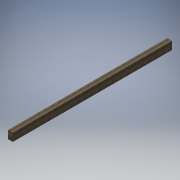
# Autodesk Inventor part: Bodenbalken
Saved by Autodesk Inventor 2017 (Build 210142000, 142)
## iProperties
Created: 2017-05-11
Part Number: Bodenbalken
Material: Generic
Document SubType Name: Modeling
Designer: Fake
Density: 1 g/cm^3
Appearance: Treibholz
Author: Fake
Autodesk Inventor part; units mm, degrees
ref_plane "YZ Plane" through (0, 0, 0) normal (1, 0, 0) x (0, 1, 0)
ref_plane "XZ Plane" through (0, 0, 0) normal (0, 1, 0) x (-1, 0, 0)
ref_plane "XY Plane" through (0, 0, 0) normal (0, 0, 1) x (1, 0, 0)
sketch "Skizze2" plane through (0, 0, 0) normal (0, 1, 0) x (-1, 0, 0)
  line L0 (30, 50) -> (-30, 50)
  line L1 (-30, 50) -> (-30, -50)
  line L2 (-30, -50) -> (30, -50)
  line L3 (30, -50) -> (30, 50)
  line L4 (0, -70) -> (0, 70) projected
  line L5 (42, 0) -> (-42, 0) projected
  dimension "d2" = 60
  dimension "d3" = 100
  constraints: 8 end point, 2 parallel, 1 horizontal, 1 perpendicular, 2 other
  measures "d2" distance of L0.start L0.end
  measures "d3" distance of L2.end L0.start
extrude "Extrusion1" add sketch "Skizze2" along normal blind 2000
